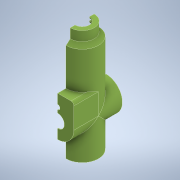
# Autodesk Inventor part: Shell V2
Saved by Autodesk Inventor 2022 (Build 260153000, 153)
## iProperties
Created: 2023-01-27
Part Number: Shell V2
Material: Generic
Document SubType Name: Modeling
Designer: ASUS
Density: 1 g/cm^3
Appearance: Olive Green
Author: ASUS
Autodesk Inventor part; units mm, degrees
ref_plane "YZ Plane" through (0, 0, 0) normal (1, 0, 0) x (0, 1, 0)
ref_plane "XZ Plane" through (0, 0, 0) normal (0, 1, 0) x (-1, 0, 0)
sketch "Sketch1" plane through (0, 0, 0) normal (0, 1, 0) x (-1, 0, 0)
  circle A0 centre (0, 0) radius 31.5
  circle A1 centre (0, 0) radius 34
  dimension "d0" = 63
  dimension "d1" = 68
  constraints: 2 centre point, 2 coincident
  measures "d0" diameter of A0
  measures "d1" diameter of A1
extrude "Extrusion1" add sketch "Sketch1" along normal blind 155.4 and the other way blind 50
ref_plane "Work Plane1" through (0, 162.9, 0) normal (0, 1, 0) x (1, 0, 0)
sketch "Sketch4" plane through (0, 0, 0) normal (1, 0, 0) x (0, 1, 0)
  line L0 (162.9, 25) -> (162.9, -25) construction
  line L1 (155.4, -34) -> (155.4, 34) projected
  line L2 (0, 0) -> (-17.0937, 0)
  line L3 (155.4, -34) -> (162.9, -25)
  line L4 (162.9, -25) -> (182.9, -25)
  line L5 (182.9, -25) -> (182.9, -23.5)
  line L6 (182.9, -23.5) -> (162.9, -23.5)
  line L7 (162.9, -23.5) -> (155.4, -32.5)
  dimension "d7" = 7.5
  dimension "d8" = 50
  dimension "d9" = 25
  dimension "d11" = 20
  dimension "d12" = 1.5
  constraints: 14 end point, 2 horizontal, 1 perpendicular, 1 point on line, 1 vertical
  measures "d7" distance between parallel lines of L1 L0
  measures "d8" distance of L0.start L0.end
  measures "d9" distance from line of L0.end L2
  measures "d11" distance of L0.end L4.end
  measures "d12" distance of L4.end L5.end
revolve "Revolution1" add sketch "Sketch4" angle 360 about axis through (0, 0, 0) along (0, -1, 0)
sketch "Sketch11" plane through (0, 0, 0) normal (1, 0, 0) x (0, 1, 0)
  line L0 (187.8356, 0) -> (132.593, 0) construction
  line L1 (162.8981, 23.5) -> (155.4, 32.5)
  line L2 (155.4, 32.5) -> (155.4, 23.5)
  line L3 (162.9, 23.5) -> (155.4, 23.5)
  line L4 (150.4, 32.5) -> (145.4, 32.5)
  line L5 (145.4, 32.5) -> (145.4, 23.8843)
  line L6 (145.4, 23.8843) -> (150.4, 23.8843)
  line L7 (150.4, 23.8843) -> (150.4, 32.5)
  point P0 (0, 0)
  dimension "d124" = 5
  dimension "d125" = 5
  constraints: 16 end point, 2 horizontal, 2 parallel, 1 perpendicular
  measures "d124" distance of L6.end L5.end
  measures "d125" distance between parallel lines of L2 L7
revolve "Revolution3" add sketch "Sketch11" angle 360 about axis through (0, 187.8356, 0) along (0, -1, 0)
sketch "Sketch12" plane through (0, 0, 0) normal (0, 0, 1) x (1, 0, 0)
  circle A0 centre (0, 27.5) radius 34
  circle A1 centre (0, 27.5) radius 32.5
  line L0 (25, 182.9) -> (-25, 182.9) projected
  point P0 (0, 0)
  dimension "d53" = 155.4
  constraints: 2 centre point, 1 coincident
  measures "d53" distance from line of L0 A0.centre
extrude "Extrusion6" add sketch "Sketch12" against normal blind 50
sketch "Sketch13" plane through (0, 0, 0) normal (0, 0, 1) x (1, 0, 0)
  arc A0 (-32.5, 27.5) -> (32.5, 27.5) centre (0, 27.5) ccw projected
  circle A1 centre (0, 27.5) radius 32.5
  point P0 (0, 0)
  point P1 (32.5, 27.5)
  constraints: 1 centre point, 1 coincident
extrude "Extrusion7" cut sketch "Sketch13" against normal blind 50
sketch "Sketch14" plane through (0, 0, 0) normal (0, 1, 0) x (-1, 0, 0)
  circle A0 centre (0, 0) radius 31
  dimension "d58" = 62
  constraints: 1 centre point, 1 coincident
  measures "d58" diameter of A0
extrude "Extrusion8" cut sketch "Sketch14" along normal blind 100 and the other way blind 40
ref_plane "Work Plane2" through (0, 27.5, -15) normal (0, 0, 1) x (-1, 0, 0)
sketch "Sketch19" plane through (0, 0, 0) normal (0, 0, 1) x (1, 0, 0)
  arc A0 (-32.5, 27.5) -> (32.5, 27.5) centre (0, 27.5) ccw
  arc A1 (-34, 27.5) -> (34, 27.5) centre (0, 27.5) ccw
  line L0 (34, 27.5) -> (34, 71.5)
  line L1 (28, 77.5) -> (-28, 77.5)
  line L2 (-34, 71.5) -> (-34, 27.5)
  arc A2 (-28, 77.5) -> (-34, 71.5) centre (-28, 71.5) ccw
  arc A3 (34, 71.5) -> (28, 77.5) centre (28, 71.5) ccw
  line L3 (-32.5, 27.5) -> (-32.5, 71.5)
  arc A4 (-28, 76) -> (-32.5, 71.5) centre (-28, 71.5) ccw
  line L4 (-28, 76) -> (28, 76)
  arc A5 (32.5, 71.5) -> (28, 76) centre (28, 71.5) ccw
  line L5 (32.5, 71.5) -> (32.5, 27.5)
  point P0 (0, 0)
  point P1 (-34, 77.5)
  point P2 (32.5, 27.5)
  dimension "d77" = 50
  dimension "d78" = 6
  dimension "d79" = 1.5
  constraints: 12 end point, 12 point on circle, 6 centre point, 4 tangent, 2 coincident, 2 parallel, 2 point on line, 1 equal radius, 4 other
  measures "d77" distance of point (-34, 77.5) L2.end
  measures "d78" radius of A2
  measures "d79" distance between parallel lines of L1 L4
ref_plane "Work Plane3" through (0, 0, 50) normal (0, 0, 1) x (1, 0, 0)
extrude "Extrusion12" add sketch "Sketch19" along normal blind 50
extrude "Extrusion13" cut sketch "Sketch19" along normal blind 50 contours L3 A4 L4 A5 L5 A0
sketch "Sketch16" plane through (0, 27.5, -15) normal (0, 0, 1) x (-1, 0, 0)
  circle A0 centre (0, 0) radius 27.5
  circle A1 centre (0, 0) radius 31.5
  line L0 (-31.5, -127.9) -> (-31.5, -122.9) projected
  point P0 (0, 27.5)
  dimension "d72" = 55
  constraints: 2 centre point, 1 coincident, 1 tangent
  measures "d72" diameter of A0
extrude "Extrusion10" add sketch "Sketch16" against normal blind 2.5
sketch "Sketch22" plane through (0, 0, 0) normal (0, 1, 0) x (-1, 0, 0)
  circle A0 centre (0, 0) radius 31
  dimension "d91" = 62
  constraints: 1 centre point, 1 coincident
  measures "d91" diameter of A0
extrude "Extrusion14" cut sketch "Sketch22" along normal blind 100 and the other way blind 100
sketch "Sketch23" plane through (0, 0, 50) normal (0, 0, 1) x (1, 0, 0)
  circle A0 centre (0, 27.5) radius 14
  circle A1 centre (0, 52.5) radius 5
  line L0 (34, 27.6398) -> (34, 71.5)
  line L1 (28, 77.5) -> (-28, 77.5)
  line L2 (-34, 71.5) -> (-34, 27.5)
  arc A2 (-28, 77.5) -> (-34, 71.5) centre (-28, 71.5) ccw
  arc A3 (34, 71.5) -> (28, 77.5) centre (28, 71.5) ccw
  circle A4 centre (0, 27.5) radius 34
  arc A5 (-34, 27.5) -> (34, 27.5) centre (0, 27.5) ccw projected
  line L3 (-34, 27.5) -> (-34, 71.5)
  line L4 (34, 27.5) -> (34, 71.5) projected
  line L5 (34, 27.5) -> (34, 71.5)
  point P0 (0, 0)
  point P1 (-32.5, 27.5)
  point P2 (-34, 77.5)
  dimension "d96" = 28
  dimension "d99" = 10
  dimension "d102" = 50
  dimension "d103" = 6
  constraints: 10 end point, 7 tangent, 5 centre point, 5 point on circle, 2 point on line, 1 coincident, 1 collinear, 1 equal radius, 1 parallel, 1 vertical
  measures "d96" diameter of A0
  measures "d99" diameter of A1
  measures "d102" distance of point (-34, 77.5) L2.end
  measures "d103" radius of A2
extrude "Extrusion15" add sketch "Sketch23" along normal blind 1.5
ref_plane "Work Plane4" through (0, 0, 26) normal (0, 0, 1) x (1, 0, 0)
sketch "Sketch24" plane through (0, 0, 26) normal (0, 0, 1) x (1, 0, 0)
  circle A0 centre (0, 27.5) radius 7.5 construction
  circle A1 centre (0, 27.5) radius 5.28 construction
  arc A2 (-14.0904, 21.0417) -> (14.0904, 21.0417) centre (0, 27.5) ccw
  line L0 (-14.0904, 21.0417) -> (-24.0901, 42.8583)
  arc A3 (24.0901, 42.8583) -> (-24.0901, 42.8583) centre (0, 53.9) ccw
  line L1 (24.0901, 42.8583) -> (14.0904, 21.0417)
  line L2 (28, 76) -> (32.5, 71.6465)
  line L3 (32.5, 71.6465) -> (32.5, 27.5)
  line L4 (-32.5, 27.5) -> (-32.5, 71.6465)
  line L5 (-32.5, 71.6465) -> (-28.2882, 76)
  line L6 (28, 76) -> (19.5, 76)
  line L7 (19.5, 76) -> (19.5, 86)
  line L8 (19.5, 86) -> (-19.531, 86)
  line L9 (-19.531, 86) -> (-19.531, 76)
  line L10 (-28.2882, 76) -> (-19.531, 76)
  arc A4 (-32.5, 29.4539) -> (32.5, 29.4539) centre (0, 27.5) ccw
  point P0 (0, 0)
  dimension "d107" = 15
  dimension "d109" = 26.4
  dimension "d111" = 10.56
  dimension "d112" = 0
  dimension "d114" = 0
  dimension "d115" = 8.5
  dimension "d116" = 10
  constraints: 22 end point, 6 point on circle, 5 centre point, 4 coincident, 4 perpendicular, 2 point on line
  measures "d107" diameter of A0
  measures "d109" distance of A0.centre point (0, 53.9)
  measures "d111" diameter of A1
  measures "d112" horizontal distance of A0.centre point (0, 53.9)
  measures "d114" distance of A0.centre point (0, 27.5)
  measures "d115" distance of L2.start L6.end
  measures "d116" distance of L6.end L7.end
extrude "Extrusion16" add sketch "Sketch24" against normal blind 2.5
sketch "Sketch26" plane through (0, 0, 0) normal (1, 0, 0) x (0, 1, 0)
  line L0 (86, 26) -> (80.3967, 26)
  line L1 (80.3967, 26) -> (80.3967, 31.5)
  line L2 (86, 31.5) -> (86, 26)
  line L3 (1.5, 26) -> (-4, 31.5)
  line L4 (1.5, 26) -> (-5.0587, 26)
  line L5 (-5.0587, 26) -> (-10.5587, 31.5)
  line L6 (86, 31.5) -> (80.3967, 31.5)
  line L7 (-10.5587, 31.5) -> (-4, 31.5)
  point P0 (0, 0)
  point P1 (145.4, 31.5)
  point P2 (77.5, 31.5)
  point P3 (-6.5, 31.5)
  point P4 (-50, 31.5)
  dimension "d119" = 5.6033
  constraints: 16 end point, 2 horizontal, 2 parallel, 1 perpendicular
  measures "d119" distance between parallel lines of L2 L1
extrude "Extrusion17" add sketch "Sketch26" along normal up to surface round surface about axis through (0, 0, 0) along (0, 1, 0) radius 31.5 far side no
extrude "Extrusion18" add sketch "Sketch26" against normal up to surface round surface about axis through (0, 0, 0) along (0, 1, 0) radius 31.5 far side no
sketch "Sketch27" plane through (0, 0, 26) normal (0, 0, 1) x (1, 0, 0)
  line L0 (-5, 5.5) -> (5, 5.5)
  line L1 (5, 5.5) -> (5, -5.5)
  line L2 (5, -5.5) -> (-5, -5.5)
  line L3 (-5, -5.5) -> (-5, 5.5)
  line L4 (-5, 5.5) -> (5, -5.5) construction
  line L5 (5, 5.5) -> (-5, -5.5) construction
  point P0 (0, 0)
  dimension "d126" = 10
  dimension "d127" = 11
  constraints: 12 end point, 2 midpoint, 2 parallel, 1 horizontal, 1 perpendicular
  measures "d126" distance of L1.end L2.end
  measures "d127" distance of L0.end L1.end
extrude "Extrusion19" cut sketch "Sketch27" along normal mid plane 6
ref_plane "Work Plane5" through (0, 0, 9.5) normal (0, 0, 1) x (1, 0, 0)
sketch "Sketch28" plane through (0, 0, 9.5) normal (0, 0, 1) x (1, 0, 0)
  circle A0 centre (0, 27.5) radius 7.5 construction
  arc A1 (-12.7268, 21.6667) -> (12.7268, 21.6667) centre (0, 27.5) ccw
  circle A2 centre (0, 53.9) radius 21.12 construction
  circle A3 centre (0, 27.5) radius 5.28 construction
  line L0 (-22.7265, 43.4833) -> (-12.7268, 21.6667)
  line L1 (22.7265, 43.4833) -> (12.7268, 21.6667)
  arc A4 (22.7265, 43.4833) -> (-22.7265, 43.4833) centre (0, 53.9) ccw
  line L2 (32.5762, 84.7198) -> (-32.5, 84.7198)
  line L3 (-32.5, 84.7198) -> (-32.5, 3.46)
  line L4 (-32.5, 3.46) -> (32.5762, 3.46)
  line L5 (32.5762, 3.46) -> (32.5762, 84.7198)
  point P0 (0, 0)
  point P1 (0, 27.5)
  point P2 (0, 27.5)
  dimension "d131" = 15
  dimension "d132" = 28
  dimension "d133" = 26.4
  dimension "d134" = 42.24
  dimension "d135" = 10.56
  dimension "d136" = 0
  dimension "d138" = 27.5
  dimension "d139" = 0
  constraints: 12 end point, 5 centre point, 5 coincident, 4 point on circle, 4 tangent, 2 parallel, 1 horizontal, 1 perpendicular
  measures "d131" diameter of A0
  measures "d132" diameter of A1
  measures "d133" distance of A0.centre point (0, 53.9)
  measures "d134" diameter of A2
  measures "d135" diameter of A3
  measures "d136" horizontal distance of A0.centre point (0, 53.9)
  measures "d138" distance of point (0, 0) point (0, 27.5)
  measures "d139" distance of point (0, 27.5) A0.centre
extrude "Extrusion20" add sketch "Sketch28" against normal blind 2.5
sketch "Sketch30" plane through (0, 0, 0) normal (1, 0, 0) x (0, 1, 0)
  line L0 (86, 23.5) -> (80.3967, 23.5)
  line L1 (80.3967, 23.5) -> (80.3967, 7)
  line L2 (80.3967, 7) -> (86, 7)
  line L3 (86, 7) -> (86, 23.5)
  line L4 (3.46, 7) -> (6.46, 7)
  line L5 (6.46, 7) -> (6.46, 26)
  line L6 (6.46, 26) -> (3.46, 26)
  line L7 (3.46, 26) -> (3.46, 7)
  point P0 (0, 0)
  dimension "d147" = 3
  constraints: 16 end point, 4 parallel, 2 horizontal, 2 perpendicular
  measures "d147" distance of L6.end L5.end
extrude "Extrusion22" add sketch "Sketch30" along normal up to surface round surface about axis through (0, 0, 0) along (0, 1, 0) radius 31.5 far side no
extrude "Extrusion23" add sketch "Sketch30" against normal up to surface round surface about axis through (0, 0, 0) along (0, 1, 0) radius 31.5 far side no
sketch "Sketch17" plane through (0, 0, 0) normal (0, 1, 0) x (-1, 0, 0)
  line L0 (0, 74.8629) -> (71.9581, 74.8629)
  line L1 (71.9581, 74.8629) -> (71.9581, -62.1877)
  line L2 (71.9581, -62.1877) -> (0, -62.1877)
  line L3 (0, -62.1877) -> (0, 74.8629)
  point P0 (0, 0)
  constraints: 8 end point, 2 parallel, 1 horizontal, 1 perpendicular
extrude "Extrusion11" cut sketch "Sketch17" along normal through all both and the other way through all
sketch "Sketch31" plane through (19.5, 86, 23.5) normal (0, 1, 0) x (1, 0, 0)
  line L0 (11.2124, 16.5) -> (-19.5, 16.5) projected
  line L1 (-19.5, 16.5) -> (0.5, 16.5)
  line L2 (0.5, 16.5) -> (0.5, 6.2857)
  line L3 (0.5, 6.2857) -> (-19.5, 6.2857)
  line L4 (-19.5, 6.2857) -> (-19.5, 16.5)
  point P0 (-19.5, 23.5)
  point P1 (0.5, 16.5)
  dimension "d152" = 20
  constraints: 8 end point, 2 parallel, 1 horizontal, 1 perpendicular
  measures "d152" distance of L2.end L3.end
extrude "Extrusion24" cut sketch "Sketch31" against normal blind 18
sketch "Sketch32" plane through (0, 0, 0) normal (1, 0, 0) x (0, 1, 0)
  line L0 (182.9, 25) -> (180.4, 25)
  line L1 (180.4, 25) -> (180.4, 15)
  line L2 (180.4, 15) -> (182.9, 15)
  line L3 (182.9, 15) -> (182.9, 25)
  line L4 (175.4, 25) -> (172.9, 25)
  line L5 (172.9, 25) -> (172.9, 15)
  line L6 (172.9, 15) -> (175.4, 15)
  line L7 (175.4, 15) -> (175.4, 25)
  line L8 (-96.58, 0) -> (229.48, 0) projected
  point P0 (0, 0)
  dimension "d155" = 15
  dimension "d156" = 5
  dimension "d157" = 2.5
  dimension "d158" = 2.5
  constraints: 16 end point, 4 parallel, 2 horizontal, 2 perpendicular, 1 point on line
  measures "d155" distance from line of point (0, 0) L2
  measures "d156" distance between parallel lines of L7 L1
  measures "d157" distance of L0.start L0.end
  measures "d158" distance of L4.start L4.end
revolve "Revolution4" add sketch "Sketch32" angle 360 about axis through (0, -10, 0) along (0, 1, 0)
sketch "Sketch33" plane through (0, 182.9, 0) normal (0, 1, 0) x (1, 0, 0)
  line L0 (0, -25) -> (0, -34) projected
  line L1 (0, -34) -> (-73.2733, -34)
  line L2 (-73.2733, -34) -> (-73.2733, 35.7754)
  line L3 (-73.2733, 35.7754) -> (0, 35.7754)
  line L4 (0, 35.7754) -> (0, -34)
  point P0 (0, 0)
  constraints: 8 end point, 2 parallel, 1 horizontal, 1 perpendicular
extrude "Extrusion25" cut sketch "Sketch33" against normal through all
body "Solid1"
